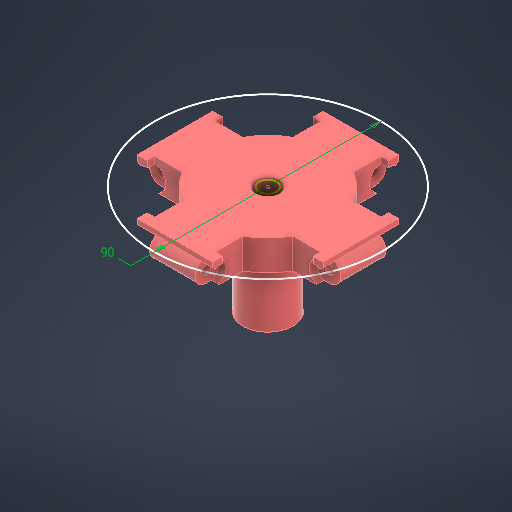
# Autodesk Inventor part: SujeccionHelices
Saved by Autodesk Inventor 2026.1 (Build 301233000, 233)
## iProperties
Created: 2025-11-10
Part Number: SujeccionHelices
Material: PLA
Document SubType Name: Modeling
Designer: vickh
Density: 1.3 g/cm^3
Appearance: Suave - Rojo
Mass: 57.6997 g
Surface Area: 138.679 cm^2
Volume: 44.3844 cm^3
Author: vickh
Autodesk Inventor part; units mm, degrees
ref_plane "YZ Plane" through (0, 0, 0) normal (1, 0, 0) x (0, 1, 0)
ref_plane "XZ Plane" through (0, 0, 0) normal (0, 1, 0) x (-1, 0, 0)
ref_plane "XY Plane" through (0, 0, 0) normal (0, 0, 1) x (1, 0, 0)
sketch "Boceto3" plane through (0, 0, 0) normal (0, 1, 0) x (-1, 0, 0)
  line L0 (-50, 50) -> (50, 50) construction
  line L1 (50, 50) -> (50, -50) construction
  line L2 (50, -50) -> (-50, -50) construction
  line L3 (-50, -50) -> (-50, 50) construction
  line L4 (-50, 50) -> (50, -50) construction
  line L5 (50, 50) -> (-50, -50) construction
  circle A0 centre (0, 0) radius 10
  dimension "d5" = 100
  dimension "d6" = 100
  dimension "d7" = 20
  constraints: 12 end point, 2 midpoint, 2 parallel, 1 centre point, 1 coincident, 1 horizontal, 1 perpendicular
  measures "d5" distance of L1.end L2.end
  measures "d6" distance of L0.end L1.end
  measures "d7" diameter of A0
extrude "Extrusión2" add sketch "Boceto3" along normal blind 31
sketch "Boceto4" plane through (0, 31, 0) normal (0, 1, 0) x (1, 0, 0)
  line L0 (-38, -12) -> (-21.9317, -12)
  line L1 (-21.9317, 12) -> (-38, 12)
  line L2 (-38, 12) -> (-38, -12)
  line L3 (-38, -12) -> (-21.9317, 12) construction
  line L4 (-21.9317, -12) -> (-38, 12) construction
  line L5 (-84.3268, 0) -> (47.4613, 0) construction
  line L6 (-12, -21.9317) -> (-12, -38)
  line L7 (-12, -38) -> (12, -38)
  line L8 (12, -38) -> (12, -21.9317)
  line L9 (21.9317, -12) -> (38, -12)
  line L10 (38, -12) -> (38, 12)
  line L11 (38, 12) -> (21.9317, 12)
  line L12 (12, 21.9317) -> (12, 38)
  line L13 (12, 38) -> (-12, 38)
  line L14 (-12, 38) -> (-12, 21.9317)
  arc A0 (21.9317, 12) -> (12, 21.9317) centre (0, 0) ccw
  arc A1 (-12, 21.9317) -> (-21.9317, 12) centre (0, 0) ccw
  arc A2 (-21.9317, -12) -> (-12, -21.9317) centre (0, 0) ccw
  arc A3 (12, -21.9317) -> (21.9317, -12) centre (0, 0) ccw
  point P0 (-29.9659, 0)
  point P1 (-29.9659, 0)
  point P2 (-38, 0)
  point P3 (-29.9659, -12)
  point P4 (0, -38)
  point P5 (12, -29.9659)
  point P6 (38, 0)
  point P7 (29.9659, 12)
  point P8 (0, 38)
  point P9 (-12, 29.9659)
  dimension "d15" = 38
  dimension "d16" = 24
  dimension "d19" = 360
  dimension "d21" = 25
  constraints: 30 end point, 8 point on circle, 5 midpoint, 4 centre point, 2 horizontal, 2 point on line, 1 coincident, 1 parallel, 1 vertical, 37 other
  measures "d15" distance of point (0, 0) point (-38, 0)
  measures "d16" distance from line of point (-29.966, -12) L1
  measures "d21" radius of A0
extrude "Extrusión3" add sketch "Boceto4" along normal blind 9
sketch "Boceto7" plane through (0, 0, 0) normal (0, -1, 0) x (1, 0, 0)
  circle A0 centre (0, 0) radius 3.45
  dimension "d26" = 6.9
  constraints: 1 centre point, 1 coincident
  measures "d26" diameter of A0
extrude "Extrusión4" cut sketch "Boceto7" against normal blind 3.5
fillet "Empalme1" radius 4.5 8 edges at (0, 31, -38) (0, 40, -38) (38, 31, 0) (38, 40, 0) (0, 31, 38) (0, 40, 38) (-38, 31, 0) (-38, 40, 0)
sketch "Boceto9" plane through (-12, 31, 21.9317) normal (-1, 0, 0) x (0, 0, 1)
  line L0 (0, 0) -> (-9.9317, 0) projected
  line L1 (0, 0) -> (16.0683, 0) construction
  line L2 (16.0683, 0) -> (16.0683, 9) construction
  line L3 (16.0683, 9) -> (0, 9) construction
  line L4 (0, 9) -> (0, 0) construction
  arc A0 (11.5683, 0) -> (11.5683, 9) centre (11.5683, 4.5) ccw construction
  line L5 (0, 9) -> (11.5683, 9) construction
  line L6 (16.0683, 9) -> (0, 0) construction
  line L7 (0, 9) -> (16.0683, 0) construction
  line L8 (0, 0) -> (0, 9) construction
  line L9 (0, 4.5) -> (16.0683, 4.5) construction
  circle A1 centre (11.5683, 4.5) radius 1.75
  point P0 (-21.9317, -31)
  dimension "d31" = 3.5
  constraints: 14 end point, 2 parallel, 1 centre point, 1 coincident, 1 collinear, 1 horizontal, 1 midpoint, 1 perpendicular, 1 point on circle, 1 tangent
  measures "d31" diameter of A1
sketch "Boceto13" plane through (0, 40, 0) normal (0, 1, 0) x (1, 0, 0)
  circle A0 centre (0, 0) radius 3.45 projected
  line L0 (-33.5, -33.5) -> (33.5, -33.5)
  line L1 (33.5, -33.5) -> (33.5, 33.5)
  line L2 (33.5, 33.5) -> (-33.5, 33.5)
  line L3 (-33.5, 33.5) -> (-33.5, -33.5)
  line L4 (-33.5, -33.5) -> (33.5, 33.5) construction
  line L5 (33.5, -33.5) -> (-33.5, 33.5) construction
  line L6 (-33.5, -12) -> (-33.5, 12) projected
  line L7 (-12, 33.5) -> (12, 33.5) projected
  constraints: 12 end point, 2 collinear, 2 midpoint, 2 parallel, 1 horizontal, 1 perpendicular
sweep "Barrido1" cut profiles "Boceto9" path "Boceto13" path curves L3 L0 L1 L2
sketch "Boceto19" plane through (0, 40, 0) normal (0, 1, 0) x (1, 0, 0)
  circle A0 centre (0, 0) radius 4.75
  dimension "d63" = 9.5
  constraints: 1 centre point, 1 coincident
  measures "d63" diameter of A0
extrude "Extrusión13" cut sketch "Boceto19" against normal blind 20
sketch "Boceto22" plane through (0, 40, 0) normal (0, 1, 0) x (1, 0, 0)
  line L0 (33.5, 12) -> (21.9317, 12) projected
  line L1 (21.9317, -12) -> (33.5, -12) projected
  line L2 (33.5, 12) -> (33.5, -12) projected
  line L3 (38, -12) -> (38, 12) projected
  line L4 (36.9317, 15) -> (21.9317, 15)
  line L5 (21.9317, 15) -> (21.9317, -15)
  line L6 (21.9317, -15) -> (36.9317, -15)
  line L7 (36.9317, -15) -> (36.9317, 15)
  line L8 (21.9317, 12) -> (21.9317, -12) construction
  line L9 (21.9317, 12) -> (21.9317, -12) construction
  line L10 (21.9317, -12) -> (38, -12) construction
  line L11 (38, -12) -> (38, 12) construction
  line L12 (38, 12) -> (21.9317, 12) construction
  line L13 (21.9317, 12) -> (38, -12) construction
  line L14 (21.9317, -12) -> (38, 12) construction
  line L15 (35.9659, 15) -> (32.9659, 15)
  line L16 (32.9659, 15) -> (32.9659, -15)
  line L17 (32.9659, -15) -> (35.9659, -15)
  line L18 (35.9659, -15) -> (35.9659, 15)
  circle A0 centre (0, 0) radius 4.75 projected
  line L19 (15, 32.9659) -> (15, 35.9659)
  line L20 (15, 21.9317) -> (15, 36.9317)
  line L21 (12, 21.9317) -> (12, 38)
  line L22 (-15, 21.9317) -> (15, 21.9317)
  line L23 (12, 21.9317) -> (-12, 38) construction
  line L24 (-12, 21.9317) -> (12, 21.9317) construction
  line L25 (-12, 21.9317) -> (12, 21.9317) construction
  line L26 (12, 38) -> (-12, 38)
  line L27 (-12, 21.9317) -> (12, 38) construction
  line L28 (15, 35.9659) -> (-15, 35.9659)
  line L29 (-15, 32.9659) -> (15, 32.9659)
  line L30 (15, 36.9317) -> (-15, 36.9317)
  line L31 (-12, 38) -> (-12, 21.9317)
  line L32 (-15, 35.9659) -> (-15, 32.9659)
  line L33 (-15, 36.9317) -> (-15, 21.9317)
  line L34 (-32.9659, 15) -> (-35.9659, 15)
  line L35 (-21.9317, 15) -> (-36.9317, 15)
  line L36 (-21.9317, 12) -> (-38, 12) construction
  line L37 (-21.9317, -15) -> (-21.9317, 15)
  line L38 (-21.9317, 12) -> (-38, -12) construction
  line L39 (-21.9317, -12) -> (-21.9317, 12) construction
  line L40 (-21.9317, -12) -> (-21.9317, 12) construction
  line L41 (-38, 12) -> (-38, -12) construction
  line L42 (-21.9317, -12) -> (-38, 12) construction
  line L43 (-35.9659, 15) -> (-35.9659, -15)
  line L44 (-32.9659, -15) -> (-32.9659, 15)
  line L45 (-36.9317, 15) -> (-36.9317, -15)
  line L46 (-38, -12) -> (-21.9317, -12) construction
  line L47 (-35.9659, -15) -> (-32.9659, -15)
  line L48 (-36.9317, -15) -> (-21.9317, -15)
  line L49 (-15, -32.9659) -> (-15, -35.9659)
  line L50 (-15, -21.9317) -> (-15, -36.9317)
  line L51 (-12, -21.9317) -> (-12, -38)
  line L52 (15, -21.9317) -> (-15, -21.9317)
  line L53 (-12, -21.9317) -> (12, -38) construction
  line L54 (12, -21.9317) -> (-12, -21.9317) construction
  line L55 (12, -21.9317) -> (-12, -21.9317) construction
  line L56 (-12, -38) -> (12, -38)
  line L57 (12, -21.9317) -> (-12, -38) construction
  line L58 (-15, -35.9659) -> (15, -35.9659)
  line L59 (15, -32.9659) -> (-15, -32.9659)
  line L60 (-15, -36.9317) -> (15, -36.9317)
  line L61 (12, -38) -> (12, -21.9317)
  line L62 (15, -35.9659) -> (15, -32.9659)
  line L63 (15, -36.9317) -> (15, -21.9317)
  line L64 (12, -33.5) -> (12, -21.9317) projected
  line L65 (-12, -21.9317) -> (-12, -33.5) projected
  line L66 (-33.5, -12) -> (-21.9317, -12) projected
  line L67 (-21.9317, 12) -> (-33.5, 12) projected
  circle A1 centre (0, 0) radius 4.75 projected
  line L68 (12, -33.5) -> (12, -21.9317) projected
  arc A2 (12, -21.9317) -> (21.9317, -12) centre (0, 0) ccw projected
  line L69 (21.9317, -12) -> (33.5, -12) projected
  line L70 (33.5, 12) -> (33.5, -12) projected
  line L71 (33.5, 12) -> (21.9317, 12) projected
  arc A3 (21.9317, 12) -> (12, 21.9317) centre (0, 0) ccw projected
  line L72 (12, 21.9317) -> (12, 33.5) projected
  line L73 (-12, 33.5) -> (12, 33.5) projected
  line L74 (-12, 33.5) -> (-12, 21.9317) projected
  arc A4 (-12, 21.9317) -> (-21.9317, 12) centre (0, 0) ccw projected
  line L75 (-21.9317, 12) -> (-33.5, 12) projected
  line L76 (-33.5, -12) -> (-33.5, 12) projected
  line L77 (-33.5, -12) -> (-21.9317, -12) projected
  arc A5 (-21.9317, -12) -> (-12, -21.9317) centre (0, 0) ccw projected
  line L78 (-12, -21.9317) -> (-12, -33.5) projected
  line L79 (12, -33.5) -> (-12, -33.5) projected
  point P0 (29.4317, -15)
  point P1 (29.9659, 0)
  point P2 (29.9659, 0)
  point P3 (32.9659, 0)
  point P4 (29.9659, 0)
  point P5 (43.9977, 12)
  point P6 (43.9977, -12)
  point P7 (32.9659, 15)
  point P8 (32.9659, 12)
  point P9 (21.9317, 12)
  point P10 (21.9317, -12)
  point P11 (32.9659, -12)
  point P12 (15, 29.4317)
  point P13 (12, 33.5)
  point P14 (0, 29.9659)
  point P15 (0, 29.9659)
  point P16 (0, 32.9659)
  point P17 (0, 29.9659)
  point P18 (-12, 33.5)
  point P19 (-29.4317, 15)
  point P20 (-29.9659, 0)
  point P21 (-29.9659, 0)
  point P22 (-32.9659, 0)
  point P23 (-29.9659, 0)
  point P24 (-15, -29.4317)
  point P25 (0, -29.9659)
  point P26 (0, -29.9659)
  point P27 (0, -32.9659)
  point P28 (0, -29.9659)
  point P29 (12, -31.3206)
  point P30 (-12, -31.3206)
  point P31 (12, 32.9659)
  point P32 (-12, 32.9659)
  point P33 (-12, 21.9317)
  point P34 (12, 21.9317)
  point P35 (-43.9977, -12)
  point P36 (-43.9977, 12)
  point P37 (-32.9659, 12)
  point P38 (-32.9659, -12)
  point P39 (-21.9317, -12)
  point P40 (-21.9317, 12)
  point P41 (12, -32.9659)
  point P42 (12, -21.9317)
  point P43 (-12, -21.9317)
  point P44 (-12, -32.9659)
  point P45 (12, 21.9317)
  point P46 (12, 32.9659)
  point P47 (-12, 32.9659)
  point P48 (-12, -32.9659)
  point P49 (12, -32.9659)
  point P50 (-12, -32.9659)
  point P51 (-32.9659, 12)
  point P52 (12, -32.9659)
  dimension "d75" = 30
  dimension "d76" = 15
  dimension "d77" = 15
  dimension "d83" = 3
  dimension "d84" = 3
  dimension "d91" = 360
  constraints: 120 end point, 12 midpoint, 8 point on line, 6 collinear, 6 parallel, 4 perpendicular, 2 horizontal, 153 other
  measures "d75" distance of L6.end L4.start
  measures "d76" distance between parallel lines of L5 L7
  measures "d77" vertical distance of point (29.432, -15) point (29.966, 0)
  measures "d83" distance of L17.end L16.end
  measures "d84" distance of point (32.966, 0) point (29.966, 0)
sketch "Boceto18" plane through (12, 31, 21.9317) normal (1, 0, 0) x (0, 0, -1)
  circle A0 centre (-11.5683, 4.5) radius 1.75 projected
  circle A1 centre (55.4317, 4.5) radius 1.75 projected
  circle A2 centre (-11.5683, 4.5) radius 5
  circle A3 centre (55.4317, 4.5) radius 5
  point P0 (21.9317, -31)
  dimension "d59" = 10
  dimension "d60" = 10
  constraints: 2 centre point, 2 coincident
  measures "d59" diameter of A2
  measures "d60" diameter of A3
sketch "Boceto15" plane through (-21.9317, 31, 12) normal (0, 0, 1) x (1, 0, 0)
  circle A0 centre (-11.5683, 4.5) radius 1.75 projected
  circle A1 centre (-11.5683, 4.5) radius 5
  circle A2 centre (55.4317, 4.5) radius 1.75 projected
  circle A3 centre (55.4317, 4.5) radius 5
  point P0 (21.9317, -31)
  dimension "d47" = 10
  dimension "d54" = 10
  constraints: 2 centre point, 2 coincident
  measures "d47" diameter of A1
  measures "d54" diameter of A3
sketch "Boceto17" plane through (-12, 31, 21.9317) normal (-1, 0, 0) x (0, 0, 1)
  circle A0 centre (11.5683, 4.5) radius 1.75 projected
  circle A1 centre (-55.4317, 4.5) radius 1.75 projected
  circle A2 centre (-55.4317, 4.5) radius 5
  circle A3 centre (11.5683, 4.5) radius 5
  point P0 (-21.9317, -31)
  dimension "d55" = 10
  dimension "d56" = 10
  constraints: 2 centre point, 2 coincident
  measures "d55" diameter of A2
  measures "d56" diameter of A3
extrude "Extrusión21" add sketch "Boceto22" along normal blind 3 contours L2 L1 L16 L0 | L0 L16 L4 L18 L6 L1 L2 | L16 L1 L5 L0 | L22 L31 L29 L21 | L4 L7 L6 L18 | L61 L59 L51 L52 | L29 L31 L73 L21 | L21 L28 L19 L29 | L61 L79 L51 L59 | L59 L62 L58 L61 | L73 L31 L28 L21 | L29 L32 L28 L31 | L37 L66 L44 L67 | L51 L58 L49 L59 | L61 L58 L51 L79 | L28 L31 L30 L21 | L21 L30 L20 L28 | L67 L76 L66 L44 L47 L43 L34 | L44 L66 L76 L67 | L63 L60 L61 L58 | L61 L60 L51 L58 | L28 L33 L30 L31 | L51 L60 L50 L58 | L43 L48 L45 L35
sketch "Boceto23" plane through (21.9317, 31, -12) normal (0, 0, -1) x (-1, 0, 0)
  circle A0 centre (-11.5683, 4.5) radius 5
  circle A1 centre (55.4317, 4.5) radius 5
  point P0 (21.9317, -31)
  point P1 (-11.5683, 4.5)
  point P2 (55.4317, 4.5)
  dimension "d94" = 10
  dimension "d95" = 10
  constraints: 2 centre point, 2 coincident
  measures "d94" diameter of A0
  measures "d95" diameter of A1
extrude "Extrusión17" cut sketch "Boceto23" along normal mid plane 6
extrude "Extrusión18" cut sketch "Boceto17" along normal mid plane 6
extrude "Extrusión19" cut sketch "Boceto15" along normal mid plane 6
extrude "Extrusión20" cut sketch "Boceto18" along normal mid plane 6
sketch "Boceto24" plane through (0, 40, 0) normal (0, 1, 0) x (1, 0, 0)
  line L0 (-21.9317, 12) -> (-21.9317, -12) projected
  arc A0 (-21.9317, -12) -> (-12, -21.9317) centre (0, 0) ccw projected
  line L1 (-12, -21.9317) -> (12, -21.9317) projected
  arc A1 (12, -21.9317) -> (21.9317, -12) centre (0, 0) ccw projected
  line L2 (21.9317, -12) -> (21.9317, 12) projected
  arc A2 (21.9317, 12) -> (12, 21.9317) centre (0, 0) ccw projected
  line L3 (12, 21.9317) -> (-12, 21.9317) projected
  arc A3 (-12, 21.9317) -> (-21.9317, 12) centre (0, 0) ccw projected
  circle A4 centre (0, 0) radius 4.75 projected
extrude "Extrusión22" add sketch "Boceto24" along normal up to surface (3 mm away)
sketch "Boceto25" plane through (0, 43, 0) normal (0, 1, 0) x (1, 0, 0)
  circle A0 centre (0, 0) radius 3.45 projected
  circle A1 centre (0, 0) radius 45
  dimension "d110" = 90
  constraints: 1 centre point, 1 coincident
  measures "d110" diameter of A1
chamfer "Chaflán1" distance 1 angle 45 4 edges at (0, 40, 36.9317) (36.9317, 40, 0) (0, 40, -36.9317) (-36.9317, 40, 0)
